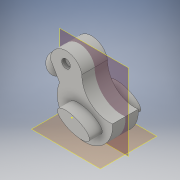
# Autodesk Inventor part: Duckhw
Saved by Autodesk Inventor 2016 (Build 200138000, 138)
## iProperties
Created: 2016-03-16
Part Number: Duckhw
Material: Generic
Document SubType Name: Modeling
Designer: Ritz
Density: 1 g/cm^3
Appearance: Default
Author: Ritz
Autodesk Inventor part; units mm, degrees
ref_plane "YZ Plane" through (0, 0, 0) normal (1, 0, 0) x (0, 1, 0)
ref_plane "XY Plane" through (0, 0, 0) normal (0, 0, 1) x (1, 0, 0)
sketch "Duck" plane through (0, 0, 0) normal (0, 0, 1) x (1, 0, 0)
  arc A0 (-0.8259, 7.3239) -> (-10.3357, 8.149) centre (-5.5831, 7.7107) ccw
  arc A1 (-0.91, 8.6813) -> (8.2069, 0.5692) centre (7.092, 8.4953) ccw
  arc A2 (-0.8338, 8.1842) -> (-0.9058, 8.1766) centre (0, 0) ccw
  arc A3 (-7.5152, 3.3464) -> (8.2069, 0.5692) centre (0, 0) ccw
  line L0 (-7.5152, 3.3464) -> (-10.3357, 8.149)
  constraints: 12 point on circle, 4 centre point, 2 end point, 1 coincident
extrude "Extrusion1" add sketch "Duck" along normal blind 7.62 contours A1 A3 L0 A0
sketch "Sketch6" plane through (0, 0, 7.62) normal (0, 0, 1) x (1, 0, 0)
  ellipse E0 centre (0.3874, -1.6659) end of major axis (5.0881, -3.3189) minor radius 2.1426
  point P0 (0, 0)
  constraints: 2 other
extrude "Extrusion3" add sketch "Sketch6" along normal blind 3.81
sketch "Sketch7" plane through (0, 0, 0) normal (0, 1, 0) x (-1, 0, 0)
  circle A0 centre (-0.4578, 3.9723) radius 1.9726
  point P0 (0, 0)
  constraints: 1 centre point
sketch "Sketch9" plane through (0, 0, 11.43) normal (0, 0, 1) x (1, 0, 0)
  point P0 (0, 0)
sketch "Sketch10" plane through (0, 0, 11.43) normal (0, 0, 1) x (1, 0, 0)
  point P0 (0, 0)
ref_plane "Work Plane8" through (0, 0, 3.81) normal (0, 0, 1) x (1, 0, 0)
mirror "Mirror6" about plane through (0, 0, 3.81) normal (0, 0, 1) of "Extrusion3"
ref_plane "Work Plane9" through (0, -8.2266, 0) normal (0, 1, 0) x (-1, 0, 0)
sketch "Sketch11" plane through (0, -8.2266, 0) normal (0, 1, 0) x (-1, 0, 0)
  circle A0 centre (0, 3.7513) radius 2.4354
  point P0 (0, 0)
  constraints: 1 centre point
extrude "Extrusion4" cut sketch "Sketch11" along normal mid plane 2.54
sketch "Sketch15" plane through (0, 0, 7.62) normal (0, 0, 1) x (1, 0, 0)
  circle A0 centre (-5.6052, 9.1445) radius 1.2764
  point P0 (0, 0)
  constraints: 1 centre point
extrude "Extrusion5" cut sketch "Sketch15" against normal blind 1
mirror "Mirror7" about plane through (0, 0, 3.81) normal (0, 0, 1) of "Extrusion5"
sketch "Sketch17" plane through (0, 0, 3.81) normal (0, 0, 1) x (1, 0, 0)
  point P0 (0, 0)
sketch "Sketch18" plane through (-7.5152, 3.3464, 0) normal (-0.8622899, -0.5064149, 0) x (0, 0, 1)
  circle A0 centre (3.8647, 2.9218) radius 1.9186
  point P0 (0, -6.6914)
  constraints: 1 centre point
extrude "Extrusion6" add sketch "Sketch18" along normal blind 4 draft 10
sketch "Sketch19" plane through (-12.444, 3.8402, 3.8647) normal (-0.8622899, -0.5064149, 0) x (0, 0, 1)
  circle A0 centre (0, 0) radius 1.5537
  point P0 (-3.8647, -9.6132)
  constraints: 1 centre point
sketch "Sketch20" plane through (-12.444, 3.8402, 3.8647) normal (-0.8622899, -0.5064149, 0) x (0, 0, 1)
  point P0 (-3.8647, -9.6132)
extrude "Extrusion7" cut sketch "Sketch19" against normal blind 5 draft 3
ref_plane "Work Plane10" through (0, 0, 3.81) normal (0, 0, 1) x (1, 0, 0)
body "Solid1"
